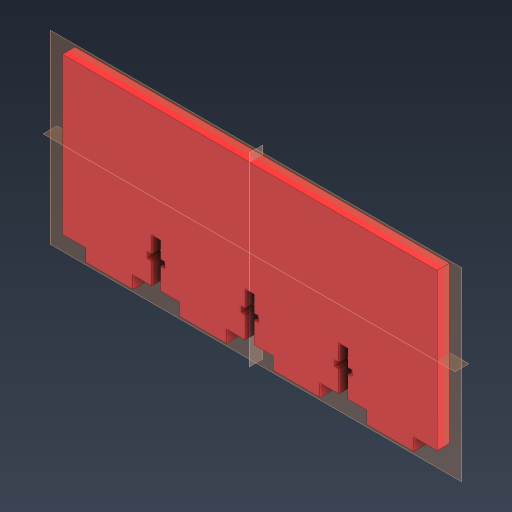
# Autodesk Inventor part: Выступ_под_крепление_маркера
Saved by Autodesk Inventor 2023.2 (Build 272271030, 271C)
## iProperties
Created: 2025-12-29
Part Number: Выступ_под_крепление_маркера
Material: Типовые
Document SubType Name: Modeling
Designer: Олег Коноваленко
Density: 1 g/cm^3
Appearance: Светло-красный
Author: Олег Коноваленко
Autodesk Inventor part; units mm, degrees
sketch "Эскиз1" plane through (0, 0, 0) normal (0, 0, 1) x (1, 0, 0)
  line L0 (-60, 25) -> (60, 25)
  line L1 (60, 25) -> (60, -25)
  line L2 (60, -25) -> (-60, -25)
  line L3 (-60, -25) -> (-60, 25)
  line L4 (-60, 25) -> (60, -25) construction
  line L5 (60, 25) -> (-60, -25) construction
  point P0 (0, 0)
  dimension "d0" = 120
  dimension "d1" = 50
  constraints: 12 end point, 2 midpoint, 2 parallel, 1 horizontal, 1 perpendicular
  measures "d0" distance of L0.start L0.end
  measures "d1" distance of L2.end L0.start
extrude "Выдавливание1" add sketch "Эскиз1" along normal mid plane 4
sketch "Эскиз2" plane through (0, 0, 2) normal (0, 0, 1) x (1, 0, 0)
  line L0 (-60, -25) -> (60, -25) projected
  line L1 (-52.5, -25) -> (-37.5, -25)
  line L2 (-37.5, -25) -> (-37.5, -29)
  line L3 (-37.5, -29) -> (-52.5, -29)
  line L4 (-52.5, -29) -> (-52.5, -25)
  line L5 (-22.5, -25) -> (-7.5, -25)
  line L6 (-7.5, -25) -> (-7.5, -29)
  line L7 (-7.5, -29) -> (-22.5, -29)
  line L8 (-22.5, -29) -> (-22.5, -25)
  line L9 (7.5, -25) -> (22.5, -25)
  line L10 (22.5, -25) -> (22.5, -29)
  line L11 (22.5, -29) -> (7.5, -29)
  line L12 (7.5, -29) -> (7.5, -25)
  line L13 (37.5, -25) -> (52.5, -25)
  line L14 (52.5, -25) -> (52.5, -29)
  line L15 (52.5, -29) -> (37.5, -29)
  line L16 (37.5, -29) -> (37.5, -25)
  point P0 (0, 0)
  dimension "d4" = 4
  dimension "d5" = 15
  dimension "d6" = 7.5
  dimension "d9" = 30
  constraints: 32 end point, 2 horizontal, 2 parallel, 1 perpendicular, 1 point on line, 24 other
  measures "d4" distance of L3.end L1.start
  measures "d5" distance of L2.end L3.end
  measures "d6" distance from line of L0.start L4
  measures "d9" distance of L1.start L5.start
extrude "Выдавливание2" add sketch "Эскиз2" against normal up to surface (4 mm away)
sketch "Эскиз3" plane through (0, 0, 2) normal (0, 0, 1) x (1, 0, 0)
  line L0 (-22.5, -25) -> (-37.5, -25) projected
  line L1 (-28.55, -25) -> (-31.45, -25)
  line L2 (-31.45, -25) -> (-31.45, -10.9)
  line L3 (-31.45, -10.9) -> (-28.55, -10.9)
  line L4 (-28.55, -10.9) -> (-28.55, -25)
  line L5 (7.5, -25) -> (-7.5, -25) projected
  line L6 (1.45, -25) -> (-1.45, -25)
  line L7 (-1.45, -25) -> (-1.45, -10.9)
  line L8 (-1.45, -10.9) -> (1.45, -10.9)
  line L9 (1.45, -10.9) -> (1.45, -25)
  line L10 (31.45, -25) -> (28.55, -25)
  line L11 (28.55, -25) -> (28.55, -10.9)
  line L12 (28.55, -10.9) -> (31.45, -10.9)
  line L13 (31.45, -10.9) -> (31.45, -25)
  line L14 (22.5, -25) -> (37.5, -25) projected
  line L15 (-32.8, -16.2) -> (-27.2, -16.2)
  line L16 (-27.2, -16.2) -> (-27.2, -18)
  line L17 (-27.2, -18) -> (-32.8, -18)
  line L18 (-32.8, -18) -> (-32.8, -16.2)
  line L19 (-2.8, -16.2) -> (2.8, -16.2)
  line L20 (2.8, -16.2) -> (2.8, -18)
  line L21 (2.8, -18) -> (-2.8, -18)
  line L22 (-2.8, -18) -> (-2.8, -16.2)
  line L23 (27.2, -16.2) -> (32.8, -16.2)
  line L24 (32.8, -16.2) -> (32.8, -18)
  line L25 (32.8, -18) -> (27.2, -18)
  line L26 (27.2, -18) -> (27.2, -16.2)
  line L27 (30, -10.9) -> (30, -25) construction
  line L28 (-30, -10.9) -> (-30, -25)
  line L29 (0, 35.8) -> (0, -39.8) projected
  point P0 (0, 0)
  point P1 (0, -25)
  point P2 (-30, -16.2)
  point P3 (0, -16.2)
  point P4 (30, -16.2)
  point P5 (28.55, -18)
  point P6 (31.45, -18)
  point P7 (31.45, -16.2)
  point P8 (28.55, -16.2)
  point P9 (1.45, -16.2)
  point P10 (-1.45, -16.2)
  point P11 (-1.45, -18)
  point P12 (1.45, -18)
  point P13 (-31.45, -18)
  point P14 (-28.55, -18)
  point P15 (-28.55, -16.2)
  point P16 (-31.45, -16.2)
  dimension "d16" = 2.9
  dimension "d17" = 14.1
  dimension "d18" = 5.6
  dimension "d19" = 1.8
  dimension "d20" = 7
  dimension "d21" = 7
  dimension "d22" = 7
  constraints: 52 end point, 13 parallel, 11 midpoint, 8 equal length, 6 horizontal, 6 perpendicular, 5 point on line, 1 vertical
  measures "d16" distance of L11.end L12.end
  measures "d17" distance of L12.end L10.start
  measures "d18" distance of L24.end L25.end
  measures "d19" distance of L23.end L24.end
  measures "d20" distance between parallel lines of L14 L25
  measures "d21" distance between parallel lines of L5 L21
  measures "d22" distance between parallel lines of L0 L17
extrude "Выдавливание3" cut sketch "Эскиз3" against normal up to next
